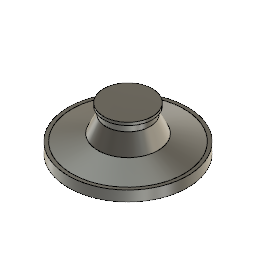
Sink_Plug (Autodesk Fusion 360 design; units mm, degrees)
Autodesk Fusion 360 part; units mm, degrees
sketch "Sketch1" plane through (0, 0, 0) normal (0, 0, 1) x (1, 0, 0)
  circle A0 centre (0, 0) radius 42.5
  dimension "d1" = 85
  measures "d1" diameter of A0
extrude "Extrude1" add sketch "Sketch1" along normal blind 7.5 makes body 1
sketch "Sketch2" plane through (0, 0, 7.5) normal (0, 0, 1) x (-1, 0, 0)
  circle A0 centre (0, 0) radius 42.5
  circle A1 centre (0, 0) radius 40
extrude "Extrude2" add sketch "Sketch2" along normal blind 5 draft -75 contours A1 bodies 1
sketch "Sketch3" plane through (0, 0, 12.5) normal (0, 0, 1) x (-1, 0, 0)
  circle A0 centre (0, 0) radius 21.3397
extrude "Extrude3" add sketch "Sketch3" along normal blind 12 draft -25 bodies 1
extrude "Extrude4" add 1 faces at (-1.9173, -4.8852, 24.5) along direction (0, 0, 1) blind 5 draft 5 on bodies 1 bodies 1
sketch "Sketch4" plane through (0, 0, 0) normal (0, 1, 0) x (1, 0, 0)
sketch "Sketch5" plane through (0, 0, 29.5) normal (0, 0, 1) x (-1, 0, 0)
  circle A0 centre (0, 0) radius 16.1815
  circle A1 centre (0, 0) radius 17.35
  dimension "d10" = 34.7
  measures "d10" diameter of A1
extrude "Extrude5" add sketch "Sketch5" along normal blind 2 separate body makes body 2
extrude "Extrude6" add 1 faces at (1.2002, -5.2586, 29.5) along direction (0, 0, 1) blind 2 on bodies 1 bodies 1 2
sketch "Sketch6" plane through (0, 0, 0) normal (0, 0, -1) x (1, 0, 0)
  circle A0 centre (0, 0) radius 42.5
  circle A1 centre (0, 0) radius 38.3224
extrude "Extrude7" cut sketch "Sketch6" against normal blind 5 contours A1 bodies 1
